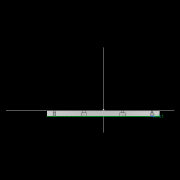
# Autodesk Inventor part: Top_Rotor_TSB
Saved by Autodesk Inventor 2022.2 (Build 262287010, 287A)
## iProperties
Created: 2022-05-21
Part Number: Top_Rotor_TSB
Material: Generic
Document SubType Name: Modeling
Designer: Árni Þór Þorgeirsson
Density: 1 g/cm^3
Appearance: Default
Author: Árni Þór Þorgeirsson
Autodesk Inventor part; units mm, degrees
ref_plane "YZ Plane" through (0, 0, 0) normal (1, 0, 0) x (0, 1, 0)
ref_plane "XZ Plane" through (0, 0, 0) normal (0, 1, 0) x (-1, 0, 0)
ref_plane "XY Plane" through (0, 0, 0) normal (0, 0, 1) x (1, 0, 0)
sketch "Sketch1" plane through (0, 0, 0) normal (0, 0, 1) x (1, 0, 0)
  circle A0 centre (0, 0) radius 14.0296 construction
  line L0 (0, 0) -> (14.0296, 0)
  line L1 (0, 0) -> (14.0296, 4.025)
  line L2 (14.0296, 0) -> (14.0296, 4.025)
  circle A1 centre (0, 0) radius 53.5
  dimension "d56" = 14.0296
  dimension "d57" = 4.025
  dimension "d400" = 53.5
  constraints: 6 end point, 2 coincident, 1 centre point, 1 horizontal, 1 horizontal alignment, 1 vertical, 4 other
  measures "d56" distance of L0.start L0.end
  measures "d57" distance of L1.end L0.end
  measures "d400" radius of A1
sketch "Sketch7" plane through (0, 0, 0) normal (0, 1, 0) x (-1, 0, 0)
  line L0 (0, 0) -> (0, 16.4739)
  line L1 (0, 0) -> (-14.0296, 0) construction
  line L2 (0, 16.4739) -> (-14.0296, 0) construction
  line L3 (0, 16.4739) -> (-19.3494, 0) construction
  line L4 (0, 16.4739) -> (-13.1819, -5.2509) construction
  line L5 (0, 0) -> (0, -16.4739)
  line L6 (0, -16.4739) -> (-14.0296, 0) construction
  line L7 (0, -16.4739) -> (-19.3494, 0) construction
  line L8 (0, -16.4739) -> (-13.1819, 5.2509) construction
  line L9 (-13.1819, 5.2509) -> (-19.3494, 0) construction
  line L10 (-9.9958, 0) -> (-19.2116, -7.8462) construction
  line L11 (-9.9958, 0) -> (-18.3269, 7.0931) construction
  line L12 (0, -30.3787) -> (0, 66.9545) projected
  line L13 (-53.5, -5.9919) -> (-53.5, 6.008)
  line L14 (15.7273, 0) -> (-94.364, 0) projected
  line L15 (-16.6891, 2.2649) -> (-11.3701, -2.2649) construction
  line L16 (-11.3701, 2.2649) -> (-16.6891, -2.2649) construction
  line L17 (-26.151, -15.9303) -> (-40.3783, -15.9303) construction
  line L18 (-40.3783, -15.9303) -> (-40.3783, -12.7539) construction
  line L19 (-40.3783, -12.7539) -> (-26.151, -12.7539) construction
  line L20 (-26.151, -12.7539) -> (-26.151, -15.9303) construction
  point P0 (-53.5, 0)
  dimension "Roller_Side_difference" = -0.015
  dimension "d90" = 16.4739
  dimension "d201" = 53.5
  dimension "d343" = 99.163
  dimension "d344" = 99.178
  dimension "d367" = 8.1
  constraints: 28 end point, 9 point on line, 3 midpoint, 3 vertical, 2 horizontal, 2 parallel, 2 perpendicular, 1 collinear, 1 symmetric about line, 2 other
  measures "d90" distance of L0.start L0.end
  measures "d201" distance between parallel lines of L5 L13
  measures "d343" angle of L10 L8
  measures "d344" angle of L7 L10
  measures "d367" distance of L3.end L8.end
sketch "Roller1" plane through (0, 0, 0) normal (0, 1, 0) x (-1, 0, 0)
  line L0 (0, 16.4739) -> (-13.1819, -5.2509) construction
  line L1 (0, 16.4739) -> (-19.3494, 0) construction
  line L2 (-9.9958, 0) -> (-18.3269, 7.0931) construction
  line L3 (0, -16.4739) -> (-19.3494, 0) construction
  line L4 (-10.0676, -0.0702) -> (-13.1486, -5.1479)
  line L5 (-13.1486, -5.1479) -> (-19.253, 0.0493)
  line L6 (-19.253, 0.0493) -> (-14.7304, 3.8997)
  line L7 (-14.7304, 3.8997) -> (-10.0676, -0.0702)
  line L8 (-12.4044, 1.9193) -> (-16.2056, -2.5453)
  line L9 (-11.643, 1.2711) -> (-15.4441, -3.1936)
  point P0 (0, 0)
  point P1 (-16.2008, -2.5493)
  dimension "d345" = 0.025
  dimension "d346" = 0.025
  dimension "d347" = 0.1
  dimension "d348" = 0.1
  dimension "d349" = 99.178
  dimension "d350" = 99.163
  dimension "d357" = 1
  dimension "d369" = 4.0148
  constraints: 12 end point, 5 parallel, 4 point on line, 1 midpoint, 1 perpendicular
  measures "d345" distance between parallel lines of L0 L4
  measures "d346" distance between parallel lines of L1 L6
  measures "d347" distance between parallel lines of L3 L5
  measures "d348" distance between parallel lines of L2 L7
  measures "d349" angle of L6 L7
  measures "d350" angle of L4 L7
  measures "d357" distance between parallel lines of L8 L9
  measures "d369" distance from line of L4.end L8
sketch "Roller2" plane through (0, 0, 0) normal (0, 1, 0) x (-1, 0, 0)
  line L0 (0, -16.4739) -> (-13.1819, 5.2509) construction
  line L1 (-9.9958, 0) -> (-19.2116, -7.8462) construction
  line L2 (0, -16.4739) -> (-19.3494, 0) construction
  line L3 (0, 16.4739) -> (-19.3494, 0) construction
  line L4 (-13.1486, 5.1479) -> (-10.0676, 0.0702)
  line L5 (-10.0676, 0.0702) -> (-14.7304, -3.8997)
  line L6 (-14.7304, -3.8997) -> (-19.253, -0.0493)
  line L7 (-19.253, -0.0493) -> (-13.1486, 5.1479)
  line L8 (-16.2008, 2.5493) -> (-12.3997, -1.9153)
  line L9 (-15.4394, 3.1976) -> (-11.6382, -1.267)
  point P0 (0, 0)
  dimension "d351" = 0.025
  dimension "d352" = 0.025
  dimension "d354" = 0.1
  dimension "d355" = 99.163
  dimension "d356" = 99.178
  dimension "d370" = 0.1
  dimension "d371" = 1
  constraints: 12 end point, 5 parallel, 3 point on line, 1 midpoint, 1 perpendicular
  measures "d351" distance between parallel lines of L0 L4
  measures "d352" distance between parallel lines of L2 L6
  measures "d354" distance between parallel lines of L1 L5
  measures "d355" angle of L5 L4
  measures "d356" angle of L6 L5
  measures "d370" distance from line of L3 L8.start
  measures "d371" distance between parallel lines of L9 L8
sketch "Sketch22" plane through (0, 0, 0) normal (0, 1, 0) x (-1, 0, 0)
  line L0 (-31.756, 8.0215) -> (-17.5287, 8.0215) construction
  line L1 (-17.5287, 8.0215) -> (-17.5287, 4.8451) construction
  line L2 (-17.5287, 4.8451) -> (-31.756, 4.8451) construction
  line L3 (-31.756, 4.8451) -> (-31.756, 8.0215) construction
  point P0 (0, 0)
  dimension "Roller_Side_difference" = -0.015
  constraints: 2 other
sketch "Sketch2" plane through (0, 0, 0) normal (0, 1, 0) x (-1, 0, 0)
  line L0 (0, 0) -> (0, 14.0296) construction
  line L1 (0, 0) -> (-14.0296, 0) projected
  line L2 (0, 0) -> (0, -14.0296)
  line L3 (0, -14.0296) -> (-14.0296, 0) construction
  line L4 (0, 14.0296) -> (-14.0296, 0) construction
  line L5 (-78.6367, 53.0497) -> (0, 14.0296) construction
  line L6 (-34.8296, 15.6811) -> (0, 14.0296) construction
  line L7 (-34.8296, 15.6811) -> (0, -14.0296) construction
  line L8 (-48.3183, 16.3206) -> (0, -14.0296) construction
  point P0 (-17.8172, -3.7876)
  constraints: 16 end point, 3 point on line, 1 perpendicular, 1 symmetric about line, 1 vertical
sketch "Sketch23" plane through (0, 0, 0) normal (0, 1, 0) x (-1, 0, 0)
  line L0 (0, -16.4739) -> (-13.1819, 5.2509) construction
  line L1 (0, -16.4739) -> (-19.3494, 0) construction
  line L2 (0, 16.4739) -> (-13.1819, -5.2509) construction
  line L3 (-13.1819, 5.2509) -> (-19.3494, 0) construction
  line L4 (0, 16.4739) -> (-19.3494, 0) construction
  line L5 (-13.1819, 5.2509) -> (-13.1819, -5.2509) construction
  line L6 (15.7273, 0) -> (-94.364, 0) projected
  line L7 (-12.1548, 3.7509) -> (-9.9103, 0.0519)
  line L8 (-9.9103, -0.0519) -> (-12.1548, -3.7509)
  line L9 (-15.098, 3.7509) -> (-19.4142, 0.0761)
  line L10 (-19.4142, -0.0761) -> (-15.098, -3.7509)
  arc A0 (-19.4142, 0.0761) -> (-19.4142, -0.0761) centre (-19.3494, 0) ccw
  arc A1 (-9.9103, -0.0519) -> (-9.9103, 0.0519) centre (-9.9958, 0) ccw
  line L11 (-12.1548, 3.7509) -> (-12.1548, 5.2509)
  line L12 (-12.1548, 5.2509) -> (-1, 5.2509)
  line L13 (-1, 5.2509) -> (-1, -5.2509)
  line L14 (-1, -5.2509) -> (-12.1548, -5.2509)
  line L15 (-12.1548, -5.2509) -> (-12.1548, -3.7509)
  line L16 (-15.098, 3.7509) -> (-15.098, 5.2509)
  line L17 (-15.098, 5.2509) -> (-53.5, 5.2509)
  line L18 (-53.5, 5.2509) -> (-53.5, -5.2509)
  line L19 (-15.098, -3.7509) -> (-15.098, -5.2509)
  line L20 (-15.098, -5.2509) -> (-53.5, -5.2509)
  line L21 (-13.1819, 5.2509) -> (-13.1819, 5.2509)
  line L22 (-13.1819, -5.2509) -> (-13.1819, -5.2509)
  line L23 (0, -30.3787) -> (0, 66.9545) projected
  line L24 (-19.5036, 0) -> (-53.5, 0)
  point P0 (0, 0)
  point P1 (-9.8788, 0)
  point P2 (-19.4494, 0)
  point P3 (-53.5, 0)
  dimension "d378" = 90
  dimension "d379" = 0.1
  dimension "d380" = 0.1
  dimension "d381" = 0.1
  dimension "d382" = 0.1
  dimension "d383" = 0.1
  dimension "d384" = 10.502
  dimension "d385" = 0
  dimension "d386" = 0
  dimension "d391" = 1
  dimension "d392" = 53.5
  dimension "d393" = 1.5
  dimension "d394" = 1.5
  dimension "d395" = 1.5
  dimension "d396" = 1.5
  constraints: 36 end point, 10 point on line, 9 vertical, 4 horizontal, 4 parallel, 4 point on circle, 4 tangent, 2 centre point, 1 equal radius, 1 midpoint
  measures "d378" angle of L6 L5
  measures "d379" radius of A0
  measures "d380" distance between parallel lines of L9 L4
  measures "d381" distance between parallel lines of L10 L1
  measures "d382" distance between parallel lines of L0 L7
  measures "d383" distance between parallel lines of L2 L8
  measures "d385" distance of L2.end L22.end
  measures "d386" distance of L0.end L21.end
  measures "d391" distance between parallel lines of L23 L13
  measures "d392" distance between parallel lines of L18 L23
  measures "d393" distance of L9.start L16.end
  measures "d394" distance of L7.start L11.end
  measures "d395" distance of L14.end L8.end
  measures "d396" distance of L10.end L19.end
revolve "RevRoller1" [suppressed]
fillet "Fillet1" [suppressed]
pattern_circular "Circular Pattern13" [suppressed]
feature "Move Body7" [suppressed]
revolve "Revolution13" [suppressed]
fillet "Fillet3" [suppressed]
pattern_circular "Circular Pattern14" [suppressed]
feature "Move Body6" [suppressed]
revolve "Revolution14" [suppressed]
revolve "OuterRim_Top2" add sketch "Sketch23" angle 360 about axis through (0, 0, -10) along (0, 0, 1) contours L6 A0 L10 L19 L20 L18
revolve "OuterRim_Bottom2" [suppressed]
extrude "Extrusion9" [suppressed]
sketch "Sketch24" plane through (0, 0, -5.251) normal (0, 0, -1) x (-1, 0, 0)
  circle A0 centre (0, 0) radius 53.5 projected
  circle A1 centre (0, 0) radius 1 projected
  line L0 (0, 0) -> (53.5, 0)
  circle A2 centre (53.5, 0) radius 1.5
  circle A3 centre (53.5, 0) radius 2.75
  point P0 (53.479, -1.4999)
  point P1 (53.479, 1.4999)
  point P2 (53.4293, -2.7491)
  point P3 (53.4293, 2.7491)
  dimension "d403" = 2.75
  dimension "d404" = 1.5
  constraints: 2 centre point, 2 coincident, 2 end point, 1 horizontal, 2 other
  measures "d403" radius of A3
  measures "d404" radius of A2
extrude "Extrusion10" [suppressed]
extrude "Extrusion11" [suppressed]
pattern_circular "Circular Pattern15" [suppressed]
sketch "Sketch25" plane through (0, 0, 5.2509) normal (0, 0, 1) x (1, 0, 0)
  circle A0 centre (-53.5, 0) radius 1.5
  line L0 (-50.8, -1.5588) -> (-53.5, -3.1177)
  line L1 (-53.5, -3.1177) -> (-56.2, -1.5588)
  line L2 (-56.2, -1.5588) -> (-56.2, 1.5588)
  line L3 (-56.2, 1.5588) -> (-53.5, 3.1177)
  line L4 (-53.5, 3.1177) -> (-50.8, 1.5588)
  line L5 (-50.8, 1.5588) -> (-50.8, -1.5588)
  arc A1 (-53.479, -1.4999) -> (-41.9314, -33.2267) centre (0, 0) ccw projected
  arc A2 (-53.479, 1.4999) -> (-53.479, -1.4999) centre (0, 0) ccw projected
  arc A3 (-41.9314, 33.2267) -> (-53.479, 1.4999) centre (0, 0) ccw projected
  circle A4 centre (0, 0) radius 1 projected
  circle A5 centre (0, 0) radius 30 construction
  circle A6 centre (0, 0) radius 45 construction
  circle A7 centre (-30, 0) radius 1.5
  circle A8 centre (-45, 0) radius 1.5
  line L6 (-32.7, 1.5588) -> (-30, 3.1177)
  line L7 (-30, 3.1177) -> (-27.3, 1.5588)
  line L8 (-27.3, 1.5588) -> (-27.3, -1.5588)
  line L9 (-27.3, -1.5588) -> (-30, -3.1177)
  line L10 (-30, -3.1177) -> (-32.7, -1.5588)
  line L11 (-32.7, -1.5588) -> (-32.7, 1.5588)
  line L12 (-47.7, 1.5588) -> (-45, 3.1177)
  line L13 (-45, 3.1177) -> (-42.3, 1.5588)
  line L14 (-42.3, 1.5588) -> (-42.3, -1.5588)
  line L15 (-42.3, -1.5588) -> (-45, -3.1177)
  line L16 (-45, -3.1177) -> (-47.7, -1.5588)
  line L17 (-47.7, -1.5588) -> (-47.7, 1.5588)
  circle A9 centre (0, 0) radius 1 projected
  line L18 (0, 0) -> (-45, 0)
  line L19 (0, 0) -> (-43.1179, -24.8941) construction
  circle A10 centre (0, 0) radius 9.9103 projected
  circle A11 centre (0, 0) radius 36.75 construction
  point P0 (-53.412, 3.0669)
  point P1 (-53.412, -3.0669)
  point P2 (-31.8264, -18.375)
  dimension "d425" = 60
  dimension "d426" = 90
  dimension "d436" = 73.5
  dimension "d412" = 5.4
  dimension "d427" = 1.5
  dimension "d428" = 1.5
  dimension "d429" = 5.4
  dimension "d430" = 5.4
  dimension "d435" = 30
  constraints: 40 end point, 8 coincident, 3 centre point, 2 horizontal alignment, 1 horizontal, 1 point on circle, 1 point on line, 46 other
  measures "d412" distance between parallel lines of L2 L5
  measures "d427" radius of A8
  measures "d428" radius of A7
  measures "d429" distance between parallel lines of L17 L14
  measures "d430" distance between parallel lines of L11 L8
  measures "d435" angle of L19 L18
extrude "Extrusion12" [suppressed]
sketch "Sketch26" plane through (0, 0, 5.251) normal (0, 0, 1) x (1, 0, 0)
  arc A0 (-53.479, 1.4999) -> (-53.479, -1.4999) centre (-53.5, 0) ccw projected
  line L0 (-56.2, 1.5588) -> (-53.5, 3.1177)
  line L1 (-53.5, 3.1177) -> (-50.8, 1.5588)
  line L2 (-50.8, 1.5588) -> (-50.8, -1.5588)
  line L3 (-50.8, -1.5588) -> (-53.5, -3.1177)
  line L4 (-53.5, -3.1177) -> (-56.2, -1.5588)
  line L5 (-56.2, -1.5588) -> (-56.2, 1.5588)
  circle A1 centre (0, 0) radius 53.5 projected
  point P0 (-53.412, -3.0669)
  point P1 (-53.412, 3.0669)
  dimension "d417" = 5.4
  constraints: 12 end point, 1 coincident, 13 other
  measures "d417" distance between parallel lines of L2 L5
extrude "Extrusion14" [suppressed]
extrude "Extrusion15" [suppressed]
pattern_circular "Circular Pattern16" [suppressed]
extrude "Extrusion16" [suppressed]
extrude "Extrusion17" [suppressed]
hole "Hole9" [suppressed]
pattern_circular "Circular Pattern17" [suppressed]
sketch "Sketch27" plane through (0, 0, -5.2509) normal (0, 0, -1) x (0, -1, 0)
  point P0 (0, 0)
  point P1 (30, 0)
  point P2 (45, 0)
  point P3 (31.8264, -18.375)
hole "Hole10" at (0, -30, -5.2509) at (0, -45, -5.2509) direction (0, 0, 1) diameter 3 depth 5.251 counterbore diameter 5.5 counterbore depth 3
hole "Hole11" at (18.375, -31.8264, -5.2509) direction (0, 0, 1) diameter 24.65 depth 5.251
pattern_circular "Circular Pattern18" count 6 over 360 about axis through (0, 0, -4.5009) along (0, 0, 1) of "Hole10", "Hole11"
extrude "Extrusion18" [suppressed]
extrude "Extrusion19" [suppressed]
pattern_circular "Circular Pattern19" [suppressed]
sketch "Sketch28" plane through (0, 0, -5.2509) normal (0, 0, -1) x (-1, 0, 0)
  circle A0 centre (0, 0) radius 53.5 projected
  circle A1 centre (46.3324, 26.75) radius 1.5
  circle A2 centre (46.3324, 26.75) radius 2.75
  circle A3 centre (38.9711, 22.5) radius 1.5 projected
  point P0 (53.5, 0)
  point P1 (45.5642, 28.0384)
  point P2 (47.0641, 25.4406)
  point P3 (44.8966, 29.0954)
  point P4 (47.6457, 24.3339)
  point P5 (42.6963, -32.2378)
  point P6 (53.4293, -2.7491)
  dimension "d472" = 1.5
  constraints: 2 centre point
  measures "d472" radius of A1
extrude "Extrusion20" cut sketch "Sketch28" against normal blind 5.251 contours A1 A0 | A0 A1
extrude "Extrusion22" cut sketch "Sketch28" against normal blind 3 contours A2 A0 A1 | A0 A1 A2
pattern_circular "Circular Pattern21" count 9 over 360 about axis through (0, 0, -4.5009) along (0, 0, 1) of "Extrusion20", "Extrusion22"
sketch "Sketch14" plane through (0, 0, -6) normal (0, 0, -1) x (-1, 0, 0)
  spline S0 degree 3 poles (-56.8, 0) (-56.8, -1.4319) (-57.0266, -2.8218) (-57.3141, -4.0377) (-57.7676, -5.9558) (-58.3249, -7.5697) (-58.7222, -9.3953) (-59.1369, -11.3012) (-59.3869, -13.435) (-59.2247, -15.7235) (-59.0417, -18.3045) (-58.3019, -21.0371) (-57.0692, -23.4317) (-55.9716, -25.5639) (-54.5147, -27.4028) (-52.9916, -28.8594) (-51.6098, -30.1808) (-50.1991, -31.1871) (-48.7772, -32.1565) (-47.6582, -32.9193) (-46.4886, -33.6761) (-45.2876, -34.7145) (-44.2461, -35.6149) (-43.2239, -36.7614) (-42.4465, -37.9481) (-41.5522, -39.3132) (-40.9615, -40.6395) (-40.4023, -41.8816) (-39.6981, -43.4458) (-39.012, -44.9714) (-38.0364, -46.5419) (-36.8523, -48.4481) (-35.229, -50.3909) (-33.1724, -51.9911) (-31.0828, -53.6171) (-28.5762, -54.8431) (-26.0987, -55.5082) (-23.9667, -56.0805) (-21.8887, -56.2534) (-19.9964, -56.2163) (-18.2263, -56.1816) (-16.6275, -55.9648) (-14.8704, -55.8135) (-13.6437, -55.7079) (-12.287, -55.6403) (-10.8418, -55.7977) (-9.4051, -55.954) (-7.9582, -56.3561) (-6.723, -56.8409) (-4.72, -57.6271) (-3.1609, -58.5239) (-1.3743, -59.2859) (0.4339, -60.0571) (2.4841, -60.7211) (4.7859, -61.008) (7.2974, -61.3212) (10.0699, -61.1458) (12.6364, -60.4279) (15.0685, -59.7477) (17.2767, -58.6047) (19.0781, -57.3063) (20.675, -56.1553) (21.9478, -54.9116) (23.1791, -53.6504) (24.0931, -52.7142) (25.0062, -51.7331) (26.1738, -50.758) (27.2513, -49.8582) (28.5815, -49.0078) (29.9203, -48.4225) (31.362, -47.7921) (32.7293, -47.438) (34.0061, -47.1128) (35.7099, -46.6787) (37.3575, -46.2745) (39.1066, -45.5849) (41.1221, -44.7903) (43.2458, -43.605) (45.1448, -41.9571) (47.1257, -40.238) (48.8124, -38.0317) (49.9482, -35.7294) (50.9787, -33.6408) (51.5623, -31.5143) (51.8755, -29.5515) (52.1638, -27.7446) (52.2245, -26.087) (52.3894, -24.2693) (52.5001, -23.0492) (52.6748, -21.7055) (53.0824, -20.3178) (53.486, -18.9435) (54.1251, -17.6047) (54.8078, -16.4847) (55.8849, -14.7175) (56.9946, -13.3786) (58.0206, -11.8296) (59.0577, -10.2638) (60.0421, -8.4781) (60.746, -6.3918) (61.5632, -3.97) (61.9524, -1.1678) (61.7393, 1.5511) (61.5477, 3.9947) (60.8853, 6.3317) (59.9849, 8.3224) (59.1769, 10.1091) (58.2036, 11.607) (57.2044, 13.0158) (56.3467, 14.2251) (55.4319, 15.3943) (54.5714, 16.8827) (53.8946, 18.0531) (53.296, 19.4496) (52.9414, 20.8302) (52.5526, 22.3437) (52.4247, 23.7538) (52.324, 25.055) (52.1844, 26.8594) (52.0852, 28.5763) (51.715, 30.453) (51.2878, 32.618) (50.4834, 34.9703) (49.1585, 37.1767) (47.7999, 39.439) (45.9031, 41.4933) (43.8164, 43.0144) (41.9871, 44.3479) (40.05, 45.273) (38.2187, 45.9151) (36.4508, 46.5351) (34.7962, 46.8888) (33.0011, 47.3754) (31.816, 47.6967) (30.5213, 48.102) (29.2246, 48.7472) (27.9361, 49.3883) (26.7251, 50.2594) (25.7377, 51.1332) (24.1248, 52.5605) (22.9654, 53.9373) (21.5425, 55.266) (20.1382, 56.5772) (18.4817, 57.8699) (16.4757, 58.9115) (14.1658, 60.1108) (11.4118, 60.9217) (8.673, 61.1141) (6.2167, 61.2866) (3.8151, 60.9744) (1.7249, 60.3891) (-0.129, 59.87) (-1.7254, 59.1596) (-3.276, 58.4164) (-4.5061, 57.8267) (-5.74, 57.1881) (-7.2319, 56.649) (-8.5094, 56.1873) (-9.9929, 55.8479) (-11.4103, 55.7465) (-12.9863, 55.6336) (-14.4057, 55.7628) (-15.7204, 55.893) (-17.5126, 56.0705) (-19.2283, 56.2635) (-21.1474, 56.213) (-23.3514, 56.155) (-25.8006, 55.7542) (-28.1882, 54.8225) (-30.6413, 53.8653) (-32.9754, 52.3479) (-34.8186, 50.5592) (-36.4742, 48.9526) (-37.7272, 47.1676) (-38.6791, 45.4442) (-39.6023, 43.7728) (-40.2354, 42.1708) (-41.0732, 40.4265) (-41.6043, 39.3209) (-42.257, 38.119) (-43.1325, 36.9822) (-43.9863, 35.8733) (-45.0213, 34.896) (-46.0149, 34.1163) (-47.6582, 32.827) (-49.1789, 31.938) (-50.7017, 30.7916) (-52.2598, 29.6185) (-53.8446, 28.1841) (-55.2311, 26.3515) (-56.7985, 24.28) (-58.0545, 21.7118) (-58.7031, 19.0595) (-59.2916, 16.6532) (-59.3854, 14.2226) (-59.1574, 12.0576) (-58.9571, 10.1553) (-58.5292, 8.4737) (-58.0655, 6.8215) (-57.7157, 5.5753) (-57.3275, 4.3132) (-57.063, 2.8386) (-56.9031, 1.9472) (-56.8, 0.9776) (-56.8, 0) knots 0 0 0 0 3.630189 3.630189 3.630189 9.356968 9.356968 9.356968 15.335248 15.335248 15.335248 22.077576 22.077576 22.077576 28.081487 28.081487 28.081487 33.527934 33.527934 33.527934 37.813991 37.813991 37.813991 41.530754 41.530754 41.530754 45.806559 45.806559 45.806559 51.191166 51.191166 51.191166 57.726747 57.726747 57.726747 64.367473 64.367473 64.367473 70.081985 70.081985 70.081985 75.427611 75.427611 75.427611 79.15967 79.15967 79.15967 82.86972 82.86972 82.86972 88.885508 88.885508 88.885508 94.974003 94.974003 94.974003 101.617247 101.617247 101.617247 107.912495 107.912495 107.912495 113.492866 113.492866 113.492866 117.63499 117.63499 117.63499 121.457377 121.457377 121.457377 125.573774 125.573774 125.573774 131.06692 131.06692 131.06692 137.396362 137.396362 137.396362 143.99916 143.99916 143.99916 149.989436 149.989436 149.989436 155.503632 155.503632 155.503632 159.204798 159.204798 159.204798 162.870082 162.870082 162.870082 168.653221 168.653221 168.653221 174.498759 174.498759 174.498759 181.284424 181.284424 181.284424 187.383433 187.383433 187.383433 192.857431 192.857431 192.857431 197.5563 197.5563 197.5563 201.251307 201.251307 201.251307 205.301831 205.301831 205.301831 210.91873 210.91873 210.91873 217.398706 217.398706 217.398706 224.043346 224.043346 224.043346 229.86837 229.86837 229.86837 235.491984 235.491984 235.491984 239.204835 239.204835 239.204835 242.894294 242.894294 242.894294 248.920758 248.920758 248.920758 254.86843 254.86843 254.86843 261.717359 261.717359 261.717359 267.860024 267.860024 267.860024 273.30815 273.30815 273.30815 277.630663 277.630663 277.630663 281.332185 281.332185 281.332185 285.447681 285.447681 285.447681 291.057972 291.057972 291.057972 297.50109 297.50109 297.50109 304.120892 304.120892 304.120892 310.066772 310.066772 310.066772 315.832644 315.832644 315.832644 319.487459 319.487459 319.487459 323.052251 323.052251 323.052251 328.947474 328.947474 328.947474 334.97976 334.97976 334.97976 341.798889 341.798889 341.798889 347.985491 347.985491 347.985491 353.421408 353.421408 353.421408 357.521549 357.521549 357.521549 360 360 360 360 projected
  circle A0 centre (0, 0) radius 55.5 projected
  point P0 (-56.8, 0)
  dimension "d226" = 5.4
  dimension "d277" = 76.5
  dimension "d319" = 30
  dimension "d320" = 5.4
  dimension "d321" = 5.4
  dimension "d246" = 2.75
  dimension "d254" = 2.75
  dimension "d255" = 3
  dimension "d293" = 60
  dimension "d294" = 90
  dimension "d305" = 30
  dimension "d107" = 0.05
  dimension "d108" = 0.05
  dimension "d109" = 0.05
  dimension "d110" = 0.05
  dimension "d112" = 0.5
  dimension "d113" = 0.5
  dimension "d114" = 0.5
  dimension "d115" = 83.909
  dimension "d116" = 83.694
  dimension "d117" = 1
  dimension "d118" = 0.05
  dimension "d119" = 0.05
  dimension "d120" = 0.05
  dimension "d121" = 0.05
  dimension "d122" = 0.5
  dimension "d123" = 0.5
  dimension "d124" = 83.909
  dimension "d125" = 83.694
  dimension "d126" = 1
  dimension "d39" = 0.05
  dimension "d41" = 0.05
  dimension "d42" = 0.5
  dimension "d43" = 0.5
  dimension "d44" = 0.5
  dimension "d45" = 0.5
  dimension "d46" = 0.5
  dimension "d47" = 0.5
  dimension "d48" = 2
  dimension "d16" = 0.05
  dimension "d17" = 0.05
  dimension "d18" = 0.05
  dimension "d19" = 0.5
  dimension "d20" = 0.5
  dimension "d21" = 0.5
  dimension "d22" = 0.5
  dimension "d23" = 0.5
  dimension "d24" = 0.5
  dimension "d28" = 2
  constraints: 8 end point, 4 point on circle, 3 parallel, 3 tangent, 2 centre point, 3 other
equation "\"Roller_Side_difference\" = -0.015459deg"
equation "\"Roller_Hole_Radius\" = 1"
equation "\"Distance_To_Bearing\" = 21.63839"
body "Solid1"
body "Solid2"
body "Solid3"
body "Solid4"
body "Solid5"
